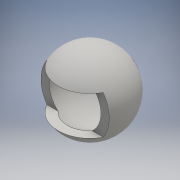
# Autodesk Inventor part: шар
Saved by Autodesk Inventor 2016 (Build 200138000, 138)
## iProperties
Created: 2016-10-19
Part Number: шар
Material: Типовые
Document SubType Name: Modeling
Designer: Student
Density: 1 g/cm^3
Appearance: По умолчанию
Mass: 22.7179 g
Surface Area: 104.585 cm^2
Volume: 22.7179 cm^3
Author: Student
Autodesk Inventor part; units mm, degrees
ref_plane "XY Plane" through (0, 0, 0) normal (0, 0, 1) x (1, 0, 0)
sketch "Эскиз1" plane through (0, 0, 0) normal (0, 0, 1) x (1, 0, 0)
  arc A0 (0, -25) -> (0, 25) centre (0, 0) ccw
  arc A1 (0, -20) -> (0, 20) centre (0, 0) ccw
  line L0 (0, 25) -> (0, 20)
  line L1 (0, -25) -> (0, -20)
  constraints: 4 end point, 4 point on circle, 2 centre point, 2 coincident, 2 point on line, 1 vertical
revolve "Вращение1" add sketch "Эскиз1" angle 360 about axis through (0, -25, 0) along (0, 1, 0)
ref_plane "РабПлоскость1" through (0, 50, 0) normal (0, 1, 0) x (-1, 0, 0)
sketch "Эскиз2" plane through (0, 50, 0) normal (0, 1, 0) x (-1, 0, 0)
  circle A0 centre (0, 0) radius 13
  dimension "d4" = 26
  constraints: 1 centre point, 1 coincident
  measures "d4" diameter of A0
extrude "Выдавливание1" cut sketch "Эскиз2" against normal blind 100
ref_plane "РабПлоскость2" through (25, 0, 0) normal (1, 0, 0) x (0, 1, 0)
sketch "Эскиз3" plane through (25, 0, 0) normal (1, 0, 0) x (0, 1, 0)
  line L0 (-10, 13) -> (-29.0962, 13)
  line L1 (-29.0962, 13) -> (-29.0962, -13)
  line L2 (-29.0962, -13) -> (-10, -13)
  line L3 (-10, -13) -> (-10, 13)
  point P0 (0, 0)
  constraints: 8 end point, 2 parallel, 1 horizontal, 1 perpendicular
extrude "Выдавливание2" cut sketch "Эскиз3" against normal blind 100
